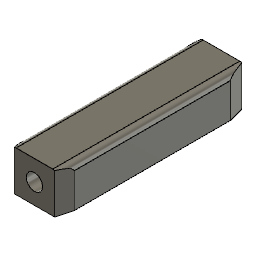
23mm Connector (Autodesk Fusion 360 archive; units mm, degrees)
design "23mm Connector"
part number: Configuration 2
Autodesk Fusion 360 part; units mm, degrees
sketch "Sketch1" plane through (0, 0, 0) normal (0, 0, 1) x (1, 0, 0)
  line L0 (3, -2.5) -> (-3, -2.5)
  line L1 (-3, -2.5) -> (-3, 2.5)
  line L2 (-3, 2.5) -> (3, 2.5)
  line L3 (3, 2.5) -> (3, -2.5)
  line L4 (3, -2.5) -> (-3, 2.5) construction
  line L5 (-3, -2.5) -> (3, 2.5) construction
  dimension "dWidth" = 6
  dimension "d2" = 5
  constraint horizontal L0
  constraint perpendicular L0 L1
  constraint parallel L0 L2
  constraint parallel L1 L3
  constraint coincident L4 origin
  constraint coincident L5 origin
  measures "dWidth" distance of L1.end L2.end
  measures "d2" distance of L0.end L1.end
extrude "Extrude1" add sketch "Sketch1" along normal blind 11.5
sketch "Sketch2" plane through (0, 0, 11.5) normal (0, 0, 1) x (1, 0, 0)
  line L0 (3, 2.5) -> (-3, 2.5)
  line L1 (-3, 2.5) -> (-3, -2.5)
  line L2 (-3, -2.5) -> (3, -2.5)
  line L3 (3, -2.5) -> (3, 2.5)
  circle A0 centre (0, 0) radius 1
  dimension "d5" = 2
  constraint coincident A0.centre origin
  measures "d5" diameter of A0
extrude "Extrude2" cut sketch "Sketch2" against normal blind 7 contours A0
ref_plane "WorkPlane1" through (0, 0, 9) normal (0, 0, 1) x (1, 0, 0)
sketch "Sketch3" plane through (0, 0, 9) normal (0, 0, 1) x (1, 0, 0)
  line L0 (2, -2.16) -> (-2, -2.16) construction
  line L1 (-2, -2.16) -> (-2, 2.16) construction
  line L2 (-2, 2.16) -> (2, 2.16) construction
  line L3 (2, 2.16) -> (2, -2.16) construction
  line L4 (2, -2.16) -> (-2, 2.16) construction
  line L5 (-2, -2.16) -> (2, 2.16) construction
  line L6 (-2, 0) -> (2, 0) construction
  line L7 (2, 1.1258) -> (2, -1.1258)
  line L8 (-2, 1.1258) -> (-2, -1.1258)
  line L9 (0, 2.16) -> (0, -2.16) construction
  line L10 (-2, 1.1258) -> (0, 2.16)
  line L11 (2, 1.1258) -> (0, 2.16)
  line L12 (-2, -1.1258) -> (0, -2.16) construction
  line L13 (0, -2.16) -> (2, -1.1258) construction
  line L14 (-2, -1.1258) -> (-2, -2.5)
  line L15 (-2, -2.5) -> (2, -2.5)
  line L16 (2, -2.5) -> (2, -1.1258)
  line L17 (3, -2.5) -> (-3, -2.5)
  dimension "d9" = 4
  dimension "d10" = 4.32
  constraint horizontal L0
  constraint perpendicular L0 L1
  constraint parallel L0 L2
  constraint parallel L1 L3
  constraint coincident L4 origin
  constraint coincident L5 origin
  constraint midpoint L1 L6.start
  constraint midpoint L3 L6.end
  constraint vertical L7
  constraint vertical L8
  constraint midpoint L6.start L8
  constraint midpoint L6.end L7
  constraint midpoint L2 L9.start
  constraint midpoint L0 L9.end
  constraint equal L7 L8
  constraint equal L8 L10
  constraint parallel L1 L14
  constraint perpendicular L14 L15
  constraint collinear L15 L17
  measures "d9" distance of L1.end L2.end
  measures "d10" distance of L0.end L1.end
extrude "Extrude3" cut sketch "Sketch3" against normal blind 1.6
fillet "Fillet1" radius 0.75 2 edges at (-3, 2.5, 5.75) (3, 2.5, 5.75)
chamfer "Chamfer2" distance 0.5 angle 75 2 edges at (3, -0.375, 11.5) (-3, -0.375, 11.5) measured on face at (-2.3296, -0.2997, 11.5) measured on face at (-2.3296, -0.2997, 11.5) tangent chain off
mirror "Mirror2" about plane through (0, 0, 0) normal (0, 0, 1) of bodies 1 merged
